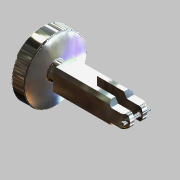
# Autodesk Inventor part: YTP-AP-E10-R1.0
Saved by Autodesk Inventor 2020.4 (Build 244396010, 396A)
## iProperties
RuleStatus: InUse
AfterDocNew0: iPropertyEnforcement
BeforeDocSave0: Materialprüfung
Created: 2021-08-29
Part Number: YTP-AP-E10-R1.0
Material: Allgemein
Document SubType Name: Modeling
Designer: Uwe Wieser
Mass: 0.377633 g
Surface Area: 5.40863 cm^2
Volume: 0.377633 cm^3
Density: 1 g/cm^3
Appearance: Chrom - poliert
Project: Airbrush
Description: Bedienhebel-Double Action
Werkstoff: 1.4301
Author: Uwe Wieser
Autodesk Inventor part; units mm, degrees
ref_plane "YZ Plane" through (0, 0, 0) normal (1, 0, 0) x (0, 1, 0)
ref_plane "XZ Plane" through (0, 0, 0) normal (0, 1, 0) x (-1, 0, 0)
ref_plane "XY Plane" through (0, 0, 0) normal (0, 0, 1) x (1, 0, 0)
sketch "Skizze1" plane through (0, 0, 0) normal (0, 0, 1) x (1, 0, 0)
  line L0 (0, 0) -> (0, 5.5)
  line L1 (0, 5.5) -> (2.5, 5.5)
  line L2 (2.5, 5.5) -> (2.5, 3)
  line L3 (4, 3) -> (17, 3)
  line L4 (17, 3) -> (17, 0)
  line L5 (17, 0) -> (0, 0)
  line L6 (-3.4, 0) -> (20.4, 0) projected
  line L7 (0, -1.1) -> (0, 6.6) projected
  line L8 (2.5, 3) -> (2.5, 1.5)
  line L9 (2.5, 1.5) -> (4, 1.5)
  line L10 (4, 1.5) -> (4, 3)
  dimension "d0" = 2.5
  dimension "d1" = 17
  dimension "d2" = 11
  dimension "d3" = 6
  dimension "d9" = 3
  dimension "d10" = 1.5
  constraints: 18 end point, 7 perpendicular, 2 point on line, 2 vertical
  measures "d0" distance of L0.end L1.end
  measures "d1" distance of L4.end L0.start
  measures "d2" diameter of L1 L6
  measures "d3" diameter of L3 L6
  measures "d9" diameter of L9 L6
  measures "d10" distance between parallel lines of L8 L10
revolve "Umdrehung1" add sketch "Skizze1" angle 360 about axis through (-10, 0, 0) along (1, 0, 0)
sketch "Skizze2" plane through (17, 0, 0) normal (1, 0, 0) x (0, 0, -1)
  circle A0 centre (0, 0) radius 3 projected
  line L0 (-2, 2) -> (2, 2)
  line L1 (2, 2) -> (2, -2)
  line L2 (2, -2) -> (-2, -2)
  line L3 (-2, -2) -> (-2, 2)
  line L4 (7.7, 0) -> (-7.7, 0) projected
  line L5 (0, -7.7) -> (0, 7.7) projected
  dimension "d5" = 4
  dimension "d6" = 4
  constraints: 8 end point, 2 parallel, 1 horizontal, 1 perpendicular, 2 other
  measures "d5" distance of L0.start L0.end
  measures "d6" distance of L0.end L1.end
extrude "Extrusion1" cut sketch "Skizze2" against normal blind 13 contours L4 L1 L0 L5 A0 | A0 L5 L2 L1 L4 | L5 L0 L3 L4 A0 | A0 L4 L3 L2 L5
sketch "Skizze3" plane through (0, 0, 0) normal (0, 0, 1) x (1, 0, 0)
  line L0 (4, -1.5) -> (4, 1.5) projected
  line L1 (-3.4, 0) -> (20.4, 0) projected
  line L2 (9, -0.75) -> (19, -0.75)
  line L3 (19, -0.75) -> (19, 0.75)
  line L4 (19, 0.75) -> (9, 0.75)
  line L5 (9, 0.75) -> (9, -0.75)
  line L6 (17, -2) -> (17, 2) projected
  point P0 (0, 0)
  dimension "d11" = 1.5
  dimension "d12" = 5
  dimension "d13" = 2
  constraints: 8 end point, 2 parallel, 1 horizontal, 1 perpendicular, 1 other
  measures "d11" distance of L4.end L2.start
  measures "d12" distance between parallel lines of L0 L5
  measures "d13" distance between parallel lines of L3 L6
extrude "Extrusion2" cut sketch "Skizze3" against normal through all both and the other way through all
fillet "Rundung1" radius 2 4 edges at (17, 1.375, 2) (17, 1.375, -2) (17, -1.375, -2) (17, -1.375, 2)
chamfer "Fase1" distance 0.5 angle 45 10 edges at (9.5, 2, 2) (16.4142, 2, 1.4142) (17, 2, 0) (16.4142, 2, -1.4142) (9.5, 2, -2) (9.5, -2, 2) (16.4142, -2, 1.4142) (16.4142, -2, -1.4142) (17, -2, 0) (9.5, -2, -2)
sketch "Skizze4" plane through (0, 0, 0) normal (0, 1, 0) x (-1, 0, 0)
  arc A0 (-15, 2) -> (-15, -2) centre (-15, 0) ccw projected
  circle A1 centre (-16.5, 0) radius 0.3
  line L0 (0, -7.7) -> (0, 7.7) projected
  line L1 (3.4112, 0) -> (-20.4019, 0) projected
  point P0 (0, 0)
  dimension "d55" = 0.6
  dimension "d56" = 16.5
  constraints: 1 centre point, 1 point on line
  measures "d55" diameter of A1
  measures "d56" distance from line of L0 A1.centre
extrude "Extrusion3" add sketch "Skizze4" along normal mid plane 5
sketch "Skizze5" plane through (0, 0, 0) normal (0, 1, 0) x (-1, 0, 0)
  line L0 (0, 5.5) -> (0, -5.5) projected
  line L1 (0, -5.5) -> (-0.2, -5.5)
  line L2 (-0.2, -5.5) -> (-0.2, 3.3)
  line L3 (-0.2, 3.3) -> (0, 3.3)
  line L4 (0, 3.3) -> (0, -5.5)
  point P0 (0, 0)
  point P1 (0, 3.3)
  dimension "d23" = 0.2
  dimension "d24" = 2.2
  constraints: 8 end point, 2 parallel, 1 horizontal, 1 perpendicular
  measures "d23" distance of L0.end L1.end
  measures "d24" distance from line of L0.start L3
extrude "Extrusion4" cut sketch "Skizze5" against normal through all both and the other way through all
fillet "Rundung2" radius 0.2 4 edges at (0.2, 0, 3.3) (0, 0, 5.5) (0.2, -1.7393, -5.2178) (0.2, 5.2178, 1.7393)
fillet "Rundung3" radius 0.2 1 edges at (2.5, -5.5, 0)
fillet "Rundung4" radius 0.2 2 edges at (2.5, -1.5, 0) (4, -1.5, 0)
sketch "Skizze6" plane through (0.2, 0, 0) normal (-1, 0, 0) x (0, 0, 1)
  line L0 (3.1, -4.1473) -> (3.1, -4.2988) projected
  line L1 (3.1, 4.1473) -> (3.1, -4.1473) projected
  line L2 (3.1, 4.2988) -> (3.1, 4.1473) projected
  arc A0 (3.1, 4.2988) -> (3.1, -4.2988) centre (0, 0) ccw projected
  arc A1 (3.1, 4.2988) -> (3.1, -4.2988) centre (0, 0) ccw projected
  line L3 (-7.7, 0) -> (7.7, 0) projected
  line L4 (-0.15, 5.2979) -> (-0.15, -5.2979)
  line L5 (0.15, -5.2979) -> (0.15, 5.2979)
  line L6 (0, -7.7) -> (0, 7.7) projected
  line L7 (0.65, -5.2979) -> (0.65, 5.2979)
  line L8 (0.35, 5.2979) -> (0.35, -5.2979)
  line L9 (1.15, -5.2979) -> (1.15, 5.2979)
  line L10 (0.85, 5.2979) -> (0.85, -5.2979)
  line L11 (1.65, -5.2979) -> (1.65, 5.2979)
  line L12 (1.35, 5.2979) -> (1.35, -5.2979)
  line L13 (2.15, -5.2979) -> (2.15, 5.2979)
  line L14 (1.85, 5.2979) -> (1.85, -5.2979)
  line L15 (2.65, -5.2979) -> (2.65, 5.2979)
  line L16 (2.35, 5.2979) -> (2.35, -5.2979)
  line L17 (3.15, -5.2979) -> (3.15, 5.2979)
  line L18 (2.85, 5.2979) -> (2.85, -5.2979)
  point P0 (0, 0)
  point P1 (2.85, 4.4685)
  point P2 (2.85, -4.4685)
  point P3 (2.35, -4.7505)
  point P4 (2.65, -4.5899)
  point P5 (2.65, 4.5899)
  point P6 (2.35, 4.7505)
  point P7 (1.85, -4.9666)
  point P8 (2.15, -4.8443)
  point P9 (2.15, 4.8443)
  point P10 (1.85, 4.9666)
  point P11 (1.35, -5.1252)
  point P12 (1.65, -5.0366)
  point P13 (1.65, 5.0366)
  point P14 (1.35, 5.1252)
  point P15 (0.85, -5.2314)
  point P16 (1.15, -5.1737)
  point P17 (1.15, 5.1737)
  point P18 (0.85, 5.2314)
  point P19 (0.35, -5.2884)
  point P20 (0.65, -5.26)
  point P21 (0.65, 5.26)
  point P22 (0.35, 5.2884)
  dimension "d35" = 0.3
  dimension "d38" = 0.5
  constraints: 28 end point, 4 point on circle, 1 horizontal, 1 vertical, 38 other
  measures "d35" distance of L4.start L5.end
  measures "d38" distance of L5.start L7.start
extrude "Extrusion5" add sketch "Skizze6" along normal blind 0.1 contours L0 A0 L18 L3 L1 | L3 L18 A0 L2 L1 | A0 L16 L3 L15 | L3 L16 A0 L15 | A0 L14 L3 L13 | L3 L14 A0 L13 | A0 L12 L3 L11 | L3 L12 A0 L11 | A0 L10 L3 L9 | L3 L10 A0 L9 | A0 L8 L3 L7 | L3 L8 A0 L7 | A0 L6 L3 L5 | L3 L6 A0 L5 | A0 L4 L3 L6 | L3 L4 A0 L6
pattern_linear "Rechteckige Anordnung1" count 11 spacing 0.5 along (0, 0, -1) of "Extrusion5"
sketch "Skizze7" plane through (0, 0, 0) normal (1, 0, 0) x (0, 1, 0)
  arc A0 (-4.2988, 3.1) -> (-4.4685, 2.85) centre (0, 0) ccw projected
  arc A1 (-4.4685, 2.85) -> (-4.5899, 2.65) centre (0, 0) ccw projected
  arc A2 (-4.5899, 2.65) -> (-4.7505, 2.35) centre (0, 0) ccw projected
  arc A3 (-4.7505, 2.35) -> (-4.8443, 2.15) centre (0, 0) ccw projected
  arc A4 (-4.8443, 2.15) -> (-4.9666, 1.85) centre (0, 0) ccw projected
  arc A5 (-4.9666, 1.85) -> (-5.0366, 1.65) centre (0, 0) ccw projected
  arc A6 (-5.0366, 1.65) -> (-5.1252, 1.35) centre (0, 0) ccw projected
  arc A7 (-5.1252, 1.35) -> (-5.1737, 1.15) centre (0, 0) ccw projected
  arc A8 (-5.1737, 1.15) -> (-5.2314, 0.85) centre (0, 0) ccw projected
  arc A9 (-5.2314, 0.85) -> (-5.26, 0.65) centre (0, 0) ccw projected
  arc A10 (-5.26, 0.65) -> (-5.2884, 0.35) centre (0, 0) ccw projected
  arc A11 (-5.2884, 0.35) -> (-5.2979, 0.15) centre (0, 0) ccw projected
  arc A12 (-5.2979, 0.15) -> (-5.2979, -0.15) centre (0, 0) ccw projected
  arc A13 (-5.2979, -0.15) -> (-5.2884, -0.35) centre (0, 0) ccw projected
  arc A14 (-5.2884, -0.35) -> (-5.26, -0.65) centre (0, 0) ccw projected
  arc A15 (-5.26, -0.65) -> (-5.2314, -0.85) centre (0, 0) ccw projected
  arc A16 (-5.2314, -0.85) -> (-5.1737, -1.15) centre (0, 0) ccw projected
  arc A17 (-5.1737, -1.15) -> (-5.1252, -1.35) centre (0, 0) ccw projected
  arc A18 (-5.1252, -1.35) -> (-5.0366, -1.65) centre (0, 0) ccw projected
  arc A19 (-5.0366, -1.65) -> (-4.9666, -1.85) centre (0, 0) ccw projected
  arc A20 (-4.9666, -1.85) -> (-4.8443, -2.15) centre (0, 0) ccw projected
  arc A21 (-4.8443, -2.15) -> (-4.7505, -2.35) centre (0, 0) ccw projected
  arc A22 (-4.7505, -2.35) -> (-4.5899, -2.65) centre (0, 0) ccw projected
  arc A23 (-4.5899, -2.65) -> (-4.4685, -2.85) centre (0, 0) ccw projected
  arc A24 (-4.4685, -2.85) -> (-4.2623, -3.15) centre (0, 0) ccw projected
  arc A25 (-4.2623, -3.15) -> (-4.107, -3.35) centre (0, 0) ccw projected
  arc A26 (-4.107, -3.35) -> (-3.8429, -3.65) centre (0, 0) ccw projected
  arc A27 (-3.8429, -3.65) -> (-3.6425, -3.85) centre (0, 0) ccw projected
  arc A28 (-3.6425, -3.85) -> (-3.2966, -4.15) centre (0, 0) ccw projected
  arc A29 (-3.2966, -4.15) -> (-3.0278, -4.35) centre (0, 0) ccw projected
  arc A30 (-3.0278, -4.35) -> (-2.5431, -4.65) centre (0, 0) ccw projected
  arc A31 (-2.5431, -4.65) -> (-2.1372, -4.85) centre (0, 0) ccw projected
  arc A32 (-2.1372, -4.85) -> (-1.252, -5.15) centre (0, 0) ccw projected
  arc A33 (-1.252, -5.15) -> (1.252, -5.15) centre (0, 0) ccw projected
  arc A34 (1.252, -5.15) -> (2.1372, -4.85) centre (0, 0) ccw projected
  arc A35 (2.1372, -4.85) -> (2.5431, -4.65) centre (0, 0) ccw projected
  arc A36 (2.5431, -4.65) -> (3.0278, -4.35) centre (0, 0) ccw projected
  arc A37 (3.0278, -4.35) -> (3.2966, -4.15) centre (0, 0) ccw projected
  arc A38 (3.2966, -4.15) -> (3.6425, -3.85) centre (0, 0) ccw projected
  arc A39 (3.6425, -3.85) -> (3.8429, -3.65) centre (0, 0) ccw projected
  arc A40 (3.8429, -3.65) -> (4.107, -3.35) centre (0, 0) ccw projected
  arc A41 (4.107, -3.35) -> (4.2623, -3.15) centre (0, 0) ccw projected
  arc A42 (4.2623, -3.15) -> (4.4685, -2.85) centre (0, 0) ccw projected
  arc A43 (4.4685, -2.85) -> (4.5899, -2.65) centre (0, 0) ccw projected
  arc A44 (4.5899, -2.65) -> (4.7505, -2.35) centre (0, 0) ccw projected
  arc A45 (4.7505, -2.35) -> (4.8443, -2.15) centre (0, 0) ccw projected
  arc A46 (4.8443, -2.15) -> (4.9666, -1.85) centre (0, 0) ccw projected
  arc A47 (4.9666, -1.85) -> (5.0366, -1.65) centre (0, 0) ccw projected
  arc A48 (5.0366, -1.65) -> (5.1252, -1.35) centre (0, 0) ccw projected
  arc A49 (5.1252, -1.35) -> (5.1737, -1.15) centre (0, 0) ccw projected
  arc A50 (5.1737, -1.15) -> (5.2314, -0.85) centre (0, 0) ccw projected
  arc A51 (5.2314, -0.85) -> (5.26, -0.65) centre (0, 0) ccw projected
  arc A52 (5.26, -0.65) -> (5.2884, -0.35) centre (0, 0) ccw projected
  arc A53 (5.2884, -0.35) -> (5.2979, -0.15) centre (0, 0) ccw projected
  arc A54 (5.2979, -0.15) -> (5.2979, 0.15) centre (0, 0) ccw projected
  arc A55 (5.2979, 0.15) -> (5.2884, 0.35) centre (0, 0) ccw projected
  arc A56 (5.2884, 0.35) -> (5.26, 0.65) centre (0, 0) ccw projected
  arc A57 (5.26, 0.65) -> (5.2314, 0.85) centre (0, 0) ccw projected
  arc A58 (5.2314, 0.85) -> (5.1737, 1.15) centre (0, 0) ccw projected
  arc A59 (5.1737, 1.15) -> (5.1252, 1.35) centre (0, 0) ccw projected
  arc A60 (5.1252, 1.35) -> (5.0366, 1.65) centre (0, 0) ccw projected
  arc A61 (5.0366, 1.65) -> (4.9666, 1.85) centre (0, 0) ccw projected
  arc A62 (4.9666, 1.85) -> (4.8443, 2.15) centre (0, 0) ccw projected
  arc A63 (4.8443, 2.15) -> (4.7505, 2.35) centre (0, 0) ccw projected
  arc A64 (4.7505, 2.35) -> (4.5899, 2.65) centre (0, 0) ccw projected
  arc A65 (4.5899, 2.65) -> (4.4685, 2.85) centre (0, 0) ccw projected
  arc A66 (4.4685, 2.85) -> (4.2988, 3.1) centre (0, 0) ccw projected
  arc A67 (-4.6155, 2.9912) -> (4.6155, 2.9912) centre (0, 0) ccw projected
  arc A68 (4.4648, 3.2118) -> (-4.4648, 3.2118) centre (0, 0) ccw projected
  line L0 (0, -10.9319) -> (0, 10.9319) projected
  line L1 (-10.9319, 0) -> (10.9319, 0) projected
  line L2 (-5.2979, -0.85) -> (5.2979, -0.85) projected
  arc A69 (-4.6155, 2.9912) -> (4.6155, 2.9912) centre (0, 0) ccw projected
  arc A70 (5.2979, -5.15) -> (5.2979, -4.85) centre (0, -5) ccw projected
  line L3 (5.2979, -5.15) -> (-5.2979, -5.15) projected
  arc A71 (-5.2979, -4.85) -> (-5.2979, -5.15) centre (0, -5) ccw projected
  line L4 (-5.2979, -4.85) -> (5.2979, -4.85) projected
  line L5 (5.2979, -4.65) -> (-5.2979, -4.65) projected
  arc A72 (-5.2979, -4.35) -> (-5.2979, -4.65) centre (0, -4.5) ccw projected
  line L6 (-5.2979, -4.35) -> (5.2979, -4.35) projected
  arc A73 (5.2979, -4.65) -> (5.2979, -4.35) centre (0, -4.5) ccw projected
  line L7 (5.2979, -4.15) -> (-5.2979, -4.15) projected
  arc A74 (-5.2979, -3.85) -> (-5.2979, -4.15) centre (0, -4) ccw projected
  line L8 (-5.2979, -3.85) -> (5.2979, -3.85) projected
  arc A75 (5.2979, -4.15) -> (5.2979, -3.85) centre (0, -4) ccw projected
  line L9 (-5.2979, -3.35) -> (5.2979, -3.35) projected
  arc A76 (5.2979, -3.65) -> (5.2979, -3.35) centre (0, -3.5) ccw projected
  line L10 (5.2979, -3.65) -> (-5.2979, -3.65) projected
  arc A77 (-5.2979, -3.35) -> (-5.2979, -3.65) centre (0, -3.5) ccw projected
  line L11 (-5.2979, -2.85) -> (5.2979, -2.85) projected
  arc A78 (5.2979, -3.15) -> (5.2979, -2.85) centre (0, -3) ccw projected
  line L12 (5.2979, -3.15) -> (-5.2979, -3.15) projected
  arc A79 (-5.2979, -2.85) -> (-5.2979, -3.15) centre (0, -3) ccw projected
  line L13 (-5.2979, -2.35) -> (5.2979, -2.35) projected
  arc A80 (5.2979, -2.65) -> (5.2979, -2.35) centre (0, -2.5) ccw projected
  line L14 (5.2979, -2.65) -> (-5.2979, -2.65) projected
  arc A81 (-5.2979, -2.35) -> (-5.2979, -2.65) centre (0, -2.5) ccw projected
  line L15 (5.2979, -2.15) -> (-5.2979, -2.15) projected
  arc A82 (-5.2979, -1.85) -> (-5.2979, -2.15) centre (0, -2) ccw projected
  line L16 (-5.2979, -1.85) -> (5.2979, -1.85) projected
  arc A83 (5.2979, -2.15) -> (5.2979, -1.85) centre (0, -2) ccw projected
  line L17 (5.2979, -1.65) -> (-5.2979, -1.65) projected
  arc A84 (-5.2979, -1.35) -> (-5.2979, -1.65) centre (0, -1.5) ccw projected
  line L18 (-5.2979, -1.35) -> (5.2979, -1.35) projected
  arc A85 (5.2979, -1.65) -> (5.2979, -1.35) centre (0, -1.5) ccw projected
  line L19 (5.2979, -1.15) -> (-5.2979, -1.15) projected
  arc A86 (-5.2979, -0.85) -> (-5.2979, -1.15) centre (0, -1) ccw projected
  line L20 (-5.2979, -0.85) -> (5.2979, -0.85) projected
  arc A87 (5.2979, -1.15) -> (5.2979, -0.85) centre (0, -1) ccw projected
  point P0 (5.1737, -1.15)
  point P1 (5.1252, -1.35)
  point P2 (5.0366, -1.65)
  point P3 (4.9666, -1.85)
  point P4 (4.8443, -2.15)
  point P5 (4.5899, -2.65)
  point P6 (4.7505, -2.35)
  point P7 (4.4685, -2.85)
  point P8 (4.2623, -3.15)
  point P9 (3.8429, -3.65)
  point P10 (4.107, -3.35)
  point P11 (3.6425, -3.85)
  point P12 (3.2966, -4.15)
  point P13 (3.0278, -4.35)
  point P14 (2.5431, -4.65)
  point P15 (2.1372, -4.85)
  point P16 (1.252, -5.15)
  point P17 (-1.252, -5.15)
  point P18 (-2.1372, -4.85)
  point P19 (-3.0278, -4.35)
  point P20 (-2.5431, -4.65)
  point P21 (-3.2966, -4.15)
  point P22 (-3.6425, -3.85)
  point P23 (-3.8429, -3.65)
  point P24 (-4.107, -3.35)
  point P25 (-4.2623, -3.15)
  point P26 (-4.4685, -2.85)
  point P27 (-4.5899, -2.65)
  point P28 (-4.7505, -2.35)
  point P29 (-4.8443, -2.15)
  point P30 (-4.9666, -1.85)
  point P31 (-5.1252, -1.35)
  point P32 (-5.0366, -1.65)
  point P33 (-5.1737, -1.15)
  constraints: 4 other
extrude "Extrusion6" cut sketch "Skizze7" along normal blind 0.2 contours A84 L18 A18 L17 A67 | A67 L17 A84 | A16 L19 A86 L2 | L2 A87 L19 A50 | L16 A20 L15 A67 | A67 L15 A82 L16 | A85 L17 A67 | A67 L17 A48 L18 A85 | L13 A22 L14 A67 | A67 L14 A81 L13 | L16 A83 L15 A67 | A67 L15 A46 L16 | L11 A24 L12 A67 | A67 L12 A79 L11 | L13 A80 L14 A67 | A67 L14 A44 L13 | L9 A26 L10 A67 | A67 L10 A77 L9 | L11 A78 L12 A67 | A67 L12 A42 L11 | L8 A28 L7 A67 | A67 L7 A74 L8 | L9 A76 L10 A67 | A67 L10 A40 L9 | L6 A30 L5 A67 | A67 L5 A72 L6 | L8 A75 L7 A67 | A67 L7 A38 L8 | L4 A32 L3 A67 | A67 L3 A71 L4 | L6 A73 L5 A67 | A67 L5 A36 L6 | L4 A70 L3 A67 | A67 L3 A34 L4
sketch "Skizze8" plane through (0, 0, 0) normal (0, 1, 0) x (-1, 0, 0)
  arc A0 (-15, 2) -> (-15, -2) centre (-15, 0) ccw projected
  line L0 (-9, 2) -> (-15, 2) projected
  line L1 (-9, -2) -> (-9, 2) projected
  line L2 (-15, -2) -> (-9, -2) projected
  arc A1 (-15, 2) -> (-15, -2) centre (-15, 0) ccw projected
  line L3 (-16.6363, 1.15) -> (-14.1907, 1.15)
  line L4 (-14.1907, 1.15) -> (-13.7, 2)
  line L5 (-9, 2) -> (-15, 2) projected
  line L6 (3.4112, 0) -> (-20.4019, 0) projected
  line L7 (-16.6363, -1.15) -> (-14.1907, -1.15)
  line L8 (-14.1907, -1.15) -> (-13.7, -2)
  point P0 (0, 0)
  dimension "d49" = 2.3
  dimension "d50" = 4.7
  dimension "d51" = 120
  constraints: 8 end point, 3 symmetric about line, 1 horizontal, 1 point on circle, 1 point on line
  measures "d49" distance of L7.start L3.start
  measures "d50" distance from line of L1 L4.end
  measures "d51" angle of L3 L4
extrude "Extrusion7" cut sketch "Skizze8" against normal through all both and the other way through all contours L0 L4 L3 A0 | L7 L8 L2 A0
fillet "Rundung7" radius 0.5 4 edges at (16.6363, -1.125, 1.15) (16.6363, 1.125, 1.15) (16.6363, -1.125, -1.15) (16.6363, 1.125, -1.15)
fillet "Rundung8" radius 0.2 8 edges at (16.2775, -2, -0.2013) (16.2775, -2, 0.2013) (16.8, 0.75, 0) (16.2775, 2, 0.2013) (16.2775, 2, -0.2013) (16.8, -0.75, 0) (16.8, -2.5, 0) (16.8, 2.5, 0)
